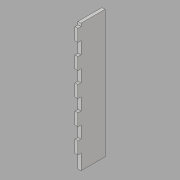
# Autodesk Inventor part: b_base_support 2
Saved by Autodesk Inventor 2019 (Build 230136000, 136)
## iProperties
Created: 2021-11-07
Part Number: b_base_support 2
Material: Generic
Document SubType Name: Modeling
Designer: Mohamed
Density: 1 g/cm^3
Appearance: Default
Author: Mohamed
Autodesk Inventor part; units mm, degrees
ref_plane "YZ Plane" through (0, 0, 0) normal (1, 0, 0) x (0, 1, 0)
ref_plane "XZ Plane" through (0, 0, 0) normal (0, 1, 0) x (-1, 0, 0)
ref_plane "XY Plane" through (0, 0, 0) normal (0, 0, 1) x (1, 0, 0)
sketch "Sketch1" plane through (0, 0, 0) normal (1, 0, 0) x (0, 1, 0)
  line L0 (33.7, 0) -> (276.7, 0)
  line L1 (283.4, -6.7) -> (283.4, -60)
  line L2 (283.4, -60) -> (0, -60)
  line L3 (0, -60) -> (0, -6.7)
  line L4 (276.7, 0) -> (276.7, -6.7)
  line L5 (276.7, -6.7) -> (283.4, -6.7)
  line L6 (33.7, 0) -> (33.7, -6.7)
  line L7 (33.7, -6.7) -> (0, -6.7)
  point P0 (0, 0)
  dimension "d0" = 283.4
  dimension "d2" = 6.7
  dimension "d3" = 6.7
  dimension "d4" = 33.7
  dimension "d5" = 6.7
  constraints: 16 end point, 2 parallel, 1 horizontal, 1 perpendicular
  measures "d0" distance of L1.end L2.end
  measures "d2" distance of L1.start L4.end
  measures "d3" distance of L0.end L4.end
  measures "d4" distance of L3.end L6.end
  measures "d5" distance of L0.start L6.end
extrude "Extrusion1" add sketch "Sketch1" along normal blind 6.7
sketch "Sketch2" plane through (6.7, 0, 0) normal (1, 0, 0) x (0, 0, -1)
  line L0 (6.7, 276.7) -> (0, 276.7) projected
  line L1 (0, 276.7) -> (0, 249.7)
  line L2 (0, 276.7) -> (0, 33.7) projected
  line L3 (0, 249.7) -> (6.7, 249.7)
  line L4 (6.7, 249.7) -> (6.7, 222.7)
  line L5 (6.7, 222.7) -> (0, 222.7)
  line L6 (0, 222.7) -> (0, 249.7)
  point P0 (0, 0)
  dimension "d8" = 27
  dimension "d9" = 6.7
  dimension "d10" = 27
  constraints: 10 end point, 2 parallel, 1 horizontal, 1 perpendicular, 1 point on line
  measures "d8" distance of L0.end L1.end
  measures "d9" distance of L4.end L5.end
  measures "d10" distance of L3.end L4.end
extrude "Extrusion2" cut sketch "Sketch2" against normal blind 6.7
pattern_linear "Rectangular Pattern1" count 4 spacing 54 along (0, -1, 0) of "Extrusion2"
body "Solid1"
